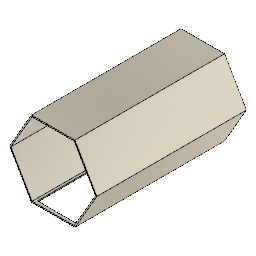
Test Fit v4 (Autodesk Fusion 360 archive; units mm, degrees)
design "dispenser box hopper"
Autodesk Fusion 360 part; units mm, degrees
sketch "side" plane through (0, 0, 0) normal (0, 1, 0) x (1, 0, 0)
  line L0 (35, -60.6218) -> (70, 0)
  line L1 (70, 0) -> (35, 60.6218)
  line L2 (35, 60.6218) -> (-35, 60.6218)
  line L3 (-35, 60.6218) -> (-70, 0)
  line L4 (-70, 0) -> (-35, -60.6218)
  line L5 (-35, -60.6218) -> (35, -60.6218)
  dimension "d1" = 70
  constraint horizontal L5
  measures "d1" distance of L0.start L4.end
extrude "Extrude1" add sketch "side" along normal blind 240
sketch "2mm offset cap" plane through (0, 0, 0) normal (0, -1, 0) x (1, 0, 0)
  line L0 (35, 60.6218) -> (-35, 60.6218)
  line L1 (-35, 60.6218) -> (-70, 0)
  line L2 (-70, 0) -> (-35, -60.6218)
  line L3 (-35, -60.6218) -> (35, -60.6218)
  line L4 (35, -60.6218) -> (70, 0)
  line L5 (70, 0) -> (35, 60.6218)
  line L6 (-35, 60.6218) -> (35, 60.6218)
  line L7 (70, 0) -> (35, 60.6218)
  line L8 (70, 0) -> (35, -60.6218)
  line L9 (35, -60.6218) -> (-35, -60.6218)
  line L10 (-35, -60.6218) -> (-70, 0)
  line L11 (-70, 0) -> (-35, 60.6218)
  line L12 (-33.8453, -58.6218) -> (-67.6906, 0)
  line L13 (-67.6906, 0) -> (-33.8453, 58.6218)
  line L14 (-33.8453, 58.6218) -> (33.8453, 58.6218)
  line L15 (67.6906, 0) -> (33.8453, 58.6218)
  line L16 (67.6906, 0) -> (33.8453, -58.6218)
  line L17 (33.8453, -58.6218) -> (-33.8453, -58.6218)
  dimension "d4" = 2
  constraint coincident L0.end L1.start
  constraint coincident L0.start L5.end
  constraint coincident L4.end L5.start
  constraint coincident L3.end L4.start
  constraint coincident L2.end L3.start
  constraint coincident L1.end L2.start
extrude "Extrude2" cut sketch "2mm offset cap" against normal blind 239 contours L12 L13 L14 L15 L16 L17
sketch "opening for tubes" plane through (0, 0, -60.6218) normal (0, 0, -1) x (1, 0, 0)
  line L0 (35, 0) -> (-35, 0)
  line L1 (-35, 0) -> (-35, -240)
  line L2 (-35, -240) -> (35, -240)
  line L3 (35, -240) -> (35, 0)
  line L4 (-35, -240) -> (35, -240)
  line L5 (35, -240) -> (35, 0)
  line L6 (35, 0) -> (-35, 0)
  line L7 (-35, 0) -> (-35, -240)
  line L8 (30, -235) -> (30, -5)
  line L9 (30, -5) -> (-30, -5)
  line L10 (-30, -5) -> (-30, -235)
  line L11 (-30, -235) -> (30, -235)
  dimension "d7" = -5
  constraint horizontal L4
  constraint vertical L5
  constraint horizontal L6
  constraint vertical L7
  constraint coincident L0.start L3.end
  constraint coincident L1.end L2.start
extrude "Extrude4" cut sketch "opening for tubes" against normal blind 2 contours L8 L9 L10 L11

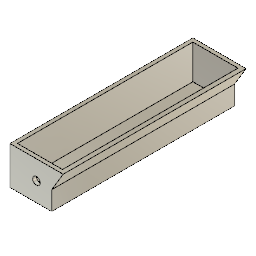
design "dispenser box tube holder"
Autodesk Fusion 360 part; units mm, degrees
sketch "side" plane through (0, 0, 0) normal (0, 1, 0) x (1, 0, 0)
  line L0 (0, 0) -> (55, 0)
  line L1 (55, 0) -> (55, -25)
  line L2 (55, -25) -> (70, -50)
  line L3 (70, -50) -> (0, -50)
  line L4 (0, -50) -> (0, 0)
  dimension "d1" = 70
  dimension "d2" = 59.036
  dimension "d3" = 50
  dimension "d4" = 25
  constraint coincident L0.start L4.end
  constraint horizontal L0
  constraint perpendicular L0 L1
  constraint perpendicular L0 L4
  constraint perpendicular L3 L4
  measures "d1" distance of L2.end L3.end
  measures "d2" angle of L2 L3
  measures "d3" distance of L3.end L0.start
  measures "d4" distance of L0.end L1.end
extrude "Extrude1" add sketch "side" along normal blind 240
shell "Shell1" thickness 5 removed faces 1 at (46.6667, 80, 50)
sketch "actuator hole" plane through (0, 0, 0) normal (0, -1, 0) x (1, 0, 0)
  line L0 (70, 50) -> (0, 50)
  line L1 (0, 50) -> (0, 0)
  line L2 (0, 0) -> (55, 0)
  line L3 (55, 0) -> (55, 25)
  line L4 (55, 25) -> (70, 50)
  circle A0 centre (35, 25) radius 5
  line L5 (35, 50) -> (35, 0)
  line L6 (0, 25) -> (15, 25)
  line L7 (15, 25) -> (55, 25)
  dimension "d8" = 10
  constraint midpoint L0 L5.start
  constraint coincident L2 L5.end
  constraint perpendicular L2 L5
  constraint coincident L1 L6.start
  constraint perpendicular L1 L6
  constraint coincident L3.end L4.start
  constraint midpoint L5 L7
  constraint midpoint A0.centre L5
  measures "d8" diameter of A0
extrude "Extrude2" cut sketch "actuator hole" against normal blind 230 contours A0 L5 L7 | A0 L5 L7 | A0 L5 L7 | A0 L5 L7

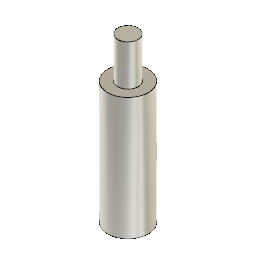
design "actuator"
Autodesk Fusion 360 part; units mm, degrees
cylinder "CylinderPrimitive1" add diameter 20 height 60 placed x (1, 0, 0) y (0, 1, 0) z (0, 0, 1) at (0, 0, 0)
sketch "cut out" plane through (0, 0, 60) normal (0, 0, 1) x (-1, 0, 0)
  circle A0 centre (0, 0) radius 10
  circle A1 centre (0, 0) radius 5
  dimension "d3" = 10
  constraint coincident A0.centre A1.centre
  measures "d3" diameter of A1
extrude "Extrude1" cut sketch "cut out" against normal blind 40 contours A1
sketch "cylinder" plane through (0, 0, 20) normal (0, 0, 1) x (-1, 0, 0)
  circle A0 centre (0, 0) radius 5
  circle A1 centre (0, 0) radius 5
  constraint coincident A0.centre A1.centre
extrude "Extrude2" add sketch "cylinder" along normal blind 60
named bodies: "actuator body"
